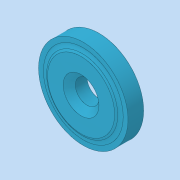
# Autodesk Inventor part: SpurGearThrustDistributer
Saved by Autodesk Inventor 2017 (Build 210142000, 142)
## iProperties
Created: 2016-11-28
Part Number: SpurGearThrustDistributer
Material: ABS Plastic
Document SubType Name: Modeling
Designer: techn
Density: 1.06 g/cm^3
Appearance: Turquoise
Author: techn
Autodesk Inventor part; units mm, degrees
ref_plane "YZ Plane" through (0, 0, 0) normal (1, 0, 0) x (0, 1, 0)
ref_plane "XZ Plane" through (0, 0, 0) normal (0, 1, 0) x (-1, 0, 0)
ref_plane "XY Plane" through (0, 0, 0) normal (0, 0, 1) x (1, 0, 0)
sketch "Sketch2" plane through (0, 0, 0) normal (0, 0, 1) x (1, 0, 0)
  circle A0 centre (0, 0) radius 4.191
  circle A1 centre (0, 0) radius 15.875
  dimension "d3" = 8.382
  dimension "d4" = 31.75
  constraints: 2 centre point, 2 coincident
  measures "d3" diameter of A0
  measures "d4" diameter of A1
extrude "Extrusion2" add sketch "Sketch2" along normal blind 6.35
sketch "Sketch3" plane through (0, 0, 0) normal (0, 0, -1) x (-1, 0, 0)
  line L0 (0, 0) -> (0, 8.3295)
  circle A0 centre (0, 8.3295) radius 4.064
  circle A1 centre (-7.2136, -4.1648) radius 4.064
  circle A2 centre (7.2136, -4.1648) radius 4.064
  dimension "d7" = 8.128
  dimension "d10" = 360
  dimension "d20" = 14.4272
  constraints: 3 centre point, 2 end point, 1 coincident, 1 vertical, 7 other
  measures "d7" diameter of A0
  measures "d20" distance of A1.centre A2.centre
extrude "Extrusion3" cut sketch "Sketch3" against normal blind 3.556
chamfer "Chamfer1" distance 2.159 angle 45 1 edges at (-4.191, 0, 6.35)
sketch "Sketch6" plane through (0, 0, 0) normal (0, 1, 0) x (-1, 0, 0)
  line L0 (15.875, 6.35) -> (-15.875, 6.35) projected
  line L1 (-15.875, 0) -> (15.875, 0) projected
  line L2 (15.875, 6.35) -> (11.9062, 6.35)
  line L3 (15.875, 6.35) -> (-15.875, 6.35) projected
  line L4 (15.875, 6.35) -> (15.875, 5.5563)
  line L5 (15.875, 0) -> (15.875, 6.35) projected
  line L6 (15.875, 5.5563) -> (13.335, 5.5563)
  line L7 (13.335, 5.5563) -> (11.9062, 6.35)
  line L8 (0, 0) -> (0, 8.967)
  dimension "d21" = 3.9688
  dimension "d22" = 0.7937
  dimension "d23" = 2.54
  constraints: 10 end point, 2 point on line, 1 perpendicular, 1 vertical
  measures "d21" distance of L0.start L2.end
  measures "d22" distance of L0.start L4.end
  measures "d23" distance of L4.end L6.end
revolve "Revolution1" cut sketch "Sketch6" angle 360 about axis through (0, 0, 0) along (0, 0, 1) contours L4 L6 L7 L0
fillet "Fillet1" radius 1.27 3 edges at (4.064, 8.3295, 3.556) (-3.1496, -4.1648, 3.556) (11.2776, -4.1648, 3.556)
fillet "Fillet2" radius 3.175 1 edges at (13.335, 0, 5.5563)
body "Solid2"
